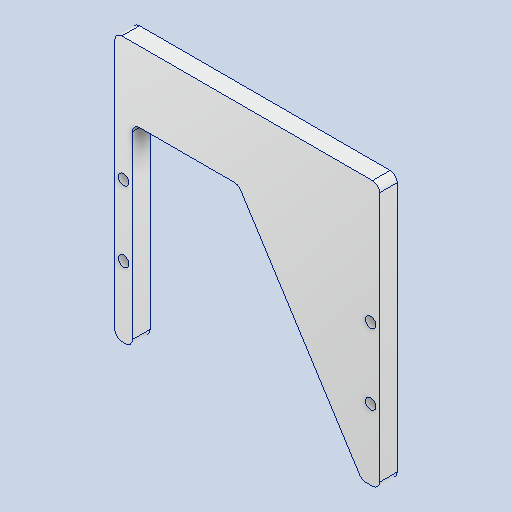
# Autodesk Inventor part: base_weel-v3-Plate-11
Saved by Autodesk Inventor 2025.2 (Build 292293000, 293)
## iProperties
Created: 2025-04-05
Part Number: base_weel-v3-Plate-11
Material: アルミニウム 6061
Document SubType Name: Modeling
Designer: haruy
Density: 2.7 g/cm^3
Appearance: アルミニウム - フラット
Author: haruy
Autodesk Inventor part; units mm, degrees
ref_plane "YZ Plane" through (0, 0, 0) normal (1, 0, 0) x (0, 1, 0)
ref_plane "XZ Plane" through (0, 0, 0) normal (0, 1, 0) x (-1, 0, 0)
ref_plane "XY Plane" through (0, 0, 0) normal (0, 0, 1) x (1, 0, 0)
derived "base_weel-v3-Plate-8.ipt"
sketch "スケッチ2" plane through (0, -355, 30) normal (0, 0, 1) x (1, 0, 0)
  line L0 (-5, 55) -> (-40, 55) projected
  line L1 (-40, 55) -> (-40, 5) projected
  line L2 (-40, 5) -> (-5, 5) projected
  line L3 (-5, 5) -> (-5, 55) projected
  line L4 (-40, 52) -> (-75, 52) projected
  line L5 (-75, 52) -> (-75, 8) projected
  line L6 (-75, 8) -> (-40, 8) projected
  line L7 (-40, 8) -> (-40, 52) projected
  line L8 (0, 0) -> (-5, 0) projected
  line L9 (-5, 0) -> (-5, 75) projected
  line L10 (0, 75) -> (-5, 75) projected
  line L11 (0, 75) -> (20, 75) projected
  line L12 (20, 75) -> (20, 55) projected
  line L13 (20, 55) -> (0, 55) projected
  line L14 (0, 55) -> (0, 75) projected
  line L15 (-75, 60) -> (-70, 60) projected
  line L16 (-70, 60) -> (-70, 0) projected
  line L17 (-70, 0) -> (-75, 0) projected
  line L18 (-75, 0) -> (-75, 60) projected
  line L19 (-5, 75) -> (-75, 75) projected
  line L20 (-75, 75) -> (-75, 55) projected
  line L21 (-75, 55) -> (-5, 55) projected
  line L22 (-5, 55) -> (-5, 75) projected
  line L23 (-5, 0) -> (-40, 55) projected
  line L24 (0, 75) -> (-5, 75) projected
  line L25 (-5, 75) -> (-5, 0) projected
  line L26 (-5, 0) -> (0, 0) projected
  line L27 (0, 0) -> (0, 75) projected
  line L28 (0, 37.5) -> (-5, 37.5) projected
  line L29 (-37.5, 75) -> (-37.5, 0) projected
  circle A0 centre (-2.5, 30) radius 1.5 projected
  circle A1 centre (-2.5, 40) radius 1.5 projected
  circle A2 centre (-2.5, 20) radius 1.5 projected
  circle A3 centre (-72.5, 40) radius 1.5 projected
  circle A4 centre (-72.5, 30) radius 1.5 projected
  circle A5 centre (-72.5, 20) radius 1.5 projected
  point P0 (0, 355)
  point P1 (0, 55)
  point P2 (-75, 60)
  point P3 (-75, 52)
  point P4 (-75, 8)
  point P5 (-70, 55)
  point P6 (-40, 55)
extrude "押し出し1" add sketch "スケッチ2" against normal blind 5 contours L3 L2 L23 L29 L0 | L9 L10 L14 L27 L28 L3 | L0 L29 L19 L9 | L29 L23 L0 | L0 L21 L16 L15 L20 L19 L29 | L28 L27 L8 L9 L3 | L9 L23 L2 | L21 L18 L15 L16 | L16 L4 L18 L21 | L16 L6 L5 L4 | L16 L17 L18 L6 | A0 | A4
fillet "フィレット1" radius 2 8 edges at (-70, -300, 27.5) (-70, -355, 27.5) (-75, -355, 27.5) (-75, -280, 27.5) (-40, -300, 27.5) (-5, -355, 27.5) (0, -355, 27.5) (0, -280, 27.5)
